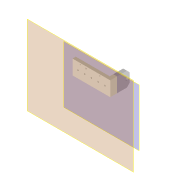
# Autodesk Inventor part: 30_XYTabel_Aliexpress_cellSTORM_xmount
Saved by Autodesk Inventor 2022 (Build 260153000, 153)
## iProperties
Created: 2021-12-30
Part Number: 30_XYTabel_Aliexpress_cellSTORM_xmount
Material: Generisch
Document SubType Name: Modeling
Designer: diederichbenedict
Density: 1 g/cm^3
Appearance: Vorgabe
Author: diederichbenedict
Autodesk Inventor part; units mm, degrees
ref_plane "YZ Plane" through (0, 0, 0) normal (1, 0, 0) x (0, 1, 0)
ref_plane "XZ Plane" through (0, 0, 0) normal (0, 1, 0) x (-1, 0, 0)
ref_plane "Arbeitsebene1" through (0, 0, 0) normal (0, 0, 1) x (1, 0, 0)
sketch "Skizze1" plane through (0, 0, 0) normal (0, 0, 1) x (1, 0, 0)
  circle A0 centre (-64.84, -24.91) radius 1.5 projected
  circle A1 centre (85.34, -22.83) radius 1 projected
  circle A2 centre (85.34, -43.41) radius 1 projected
  circle A3 centre (-64.84, 35.59) radius 1.5 projected
  circle A4 centre (-11.66, -50.59) radius 1.5 projected
  circle A5 centre (85.34, 37.77) radius 1 projected
  circle A6 centre (54.34, -50.59) radius 1.5 projected
  circle A7 centre (85.34, 58.59) radius 1 projected
  line L0 (-89.84, 67.09) -> (89.84, 67.09) projected
  line L1 (-89.84, -67.09) -> (-89.84, 67.09) projected
  line L2 (89.84, -67.09) -> (-89.84, -67.09) projected
  line L3 (89.84, 67.09) -> (89.84, -67.09) projected
  arc A8 (-32.14, 53.27) -> (-37.14, 48.27) centre (-32.14, 48.27) ccw projected
  line L4 (73.22, 53.27) -> (-32.14, 53.27) projected
  arc A9 (78.22, 48.27) -> (73.22, 53.27) centre (73.22, 48.27) ccw projected
  line L5 (78.22, -36.73) -> (78.22, 48.27) projected
  arc A10 (73.22, -41.73) -> (78.22, -36.73) centre (73.22, -36.73) ccw projected
  line L6 (-32.14, -41.73) -> (73.22, -41.73) projected
  arc A11 (-37.14, -36.73) -> (-32.14, -41.73) centre (-32.14, -36.73) ccw projected
  line L7 (-37.14, 48.27) -> (-37.14, -36.73) projected
  circle A12 centre (37.4417, 38.67) radius 1.75 projected
  circle A13 centre (24.9417, 38.67) radius 1.75 projected
  circle A14 centre (12.4417, 38.67) radius 1.75 projected
  circle A15 centre (-0.0583, 38.67) radius 1.75 projected
  line L8 (-4.46, 32.72) -> (-4.46, 44.82) construction
  line L9 (-4.46, 32.72) -> (45.54, 32.72) projected
  line L10 (45.54, 32.72) -> (45.54, 44.82) construction
  line L11 (-4.46, 44.82) -> (45.54, 44.82) projected
  circle A16 centre (36, 49.77) radius 1 projected
  circle A17 centre (10.54, 48.77) radius 1.25 projected
  line L12 (55.54, 52.32) -> (-14.46, 52.32)
  line L13 (-14.46, 52.32) -> (-14.46, 25.22)
  line L14 (-14.46, 25.22) -> (55.54, 25.22)
  line L15 (55.54, 25.22) -> (55.54, 52.32)
  circle A18 centre (20.54, 38.77) radius 1.4
  circle A19 centre (33.04, 38.77) radius 1.4
  circle A20 centre (45.54, 38.77) radius 1.4
  circle A21 centre (8.04, 38.77) radius 1.4
  circle A22 centre (20.54, 38.77) radius 1.4
  circle A23 centre (33.04, 38.77) radius 1.4
  circle A24 centre (-4.46, 38.77) radius 1.4
  circle A25 centre (8.04, 38.77) radius 1.4
  circle A26 centre (20.54, 38.77) radius 1.4
  point P0 (0, 0)
  dimension "d0" = 10
  dimension "d1" = 10
  dimension "d2" = 7.5
  dimension "d3" = 7.5
  dimension "d4" = 2.8
  dimension "d7" = 12.5
  dimension "d10" = 12.5
  constraints: 9 centre point, 8 end point, 3 horizontal, 2 parallel, 1 perpendicular, 16 other
  measures "d0" distance between parallel lines of L15 L10
  measures "d1" distance between parallel lines of L13 L8
  measures "d2" distance between parallel lines of L9 L14
  measures "d3" distance between parallel lines of L12 L11
  measures "d4" diameter of A18
  measures "d7" distance of A18.centre A19.centre
  measures "d10" distance of A18.centre A21.centre
ref_plane "Arbeitsebene2" through (-4.46, 32.72, -4) normal (0, 0, 1) x (1, 0, 0)
extrude "Extrusion1" add sketch "Skizze1" against normal blind 6 contours A12 | A13 | A14 | A15 | L15 L14 L13 L12
sketch "Skizze2" plane through (55.54, 25.22, -6) normal (0, 0, -1) x (-1, 0, 0)
  circle A0 centre (19.54, 24.55) radius 1 projected
  circle A1 centre (55.54, 24.55) radius 1 projected
  point P0 (55.54, -25.22)
hole "Bohrung1" at (0, 49.77, -6) at (36, 49.77, -6) direction (0, 0, 1) diameter 2 end through all counterbore diameter 4.5 counterbore depth 2
sketch "Skizze3" plane through (55.54, 25.22, 0) normal (1, 0, 0) x (0, 0, -1)
  line L0 (0, 27.1) -> (6, 27.1) projected
  line L1 (4, 27.1) -> (4, 0) projected
  line L2 (0, 0) -> (6, 0) projected
  line L3 (4, 0) -> (36, 0)
  line L4 (36, 0) -> (36, 27.1)
  line L5 (36, 27.1) -> (4, 27.1)
  line L6 (4, 27.1) -> (4, 0)
  circle A0 centre (31.0266, 13.55) radius 3.005 construction
  circle A1 centre (31.0266, 13.55) radius 2.8511 construction
  circle A2 centre (31.0266, 13.55) radius 2.6
  point P0 (0, -25.22)
  dimension "d22" = 32
  dimension "d44" = 5.2
  constraints: 8 end point, 2 parallel, 1 centre point, 1 horizontal, 1 perpendicular
  measures "d22" distance of L5.end L4.end
  measures "d44" diameter of A2
extrude "Extrusion2" add sketch "Skizze3" against normal blind 7
chamfer "Fase1" distance 5 angle 45 2 edges at (52.04, 52.32, -36) (52.04, 25.22, -36)
sketch "Skizze4" plane through (-14.46, 52.32, -36) normal (0, 0, -1) x (1, 0, 0)
  circle A0 centre (66.1385, 17.6805) radius 1.4
  line L0 (69.238, 10.6988) -> (61.364, 10.6988)
  line L1 (69.238, 16.4011) -> (61.364, 16.4011)
  circle A1 centre (66.1385, 9.4552) radius 1.4
  point P0 (14.46, 52.32)
  dimension "d30" = 2.8
  dimension "d41" = 2.8
  constraints: 4 end point, 2 centre point, 2 horizontal, 4 other
  measures "d30" diameter of A0
  measures "d41" diameter of A1
ref_plane "Arbeitsebene3" through (0, 0, -12.82) normal (0, 0, -1) x (-1, 0, 0)
extrude "Extrusion4" cut sketch "Skizze4" against normal blind 15
